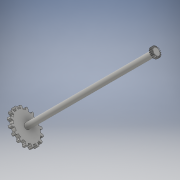
# Autodesk Inventor part: Connecting gears
Saved by Autodesk Inventor 2016 SP1 (Build 200210100, 210)
## iProperties
Created: 2016-02-23
Part Number: Connecting gears
Material: Generic
Document SubType Name: Modeling
Designer: Tore Den Store
Density: 1 g/cm^3
Appearance: Default
Author: Tore Den Store
Autodesk Inventor part; units mm, degrees
ref_plane "YZ Plane" through (0, 0, 0) normal (1, 0, 0) x (0, 1, 0)
ref_plane "XZ Plane" through (0, 0, 0) normal (0, 1, 0) x (-1, 0, 0)
ref_plane "XY Plane" through (0, 0, 0) normal (0, 0, 1) x (1, 0, 0)
sketch "Sketch1" plane through (0, 0, 0) normal (0, 1, 0) x (-1, 0, 0)
  circle A0 centre (0, 0) radius 100
  dimension "d0" = 200
  constraints: 1 centre point, 1 coincident
  measures "d0" diameter of A0
extrude "Extrusion1" add sketch "Sketch1" along normal blind 25
sketch "Sketch2" plane through (0, 25, 0) normal (0, 1, 0) x (1, 0, 0)
  circle A0 centre (0, 0) radius 100 projected
  line L0 (0, 0) -> (-99.5185, -9.8017)
  line L1 (0, 0) -> (-99.5185, 9.8017)
  line L2 (0, 0) -> (-100, 0) construction
  circle A1 centre (0, 0) radius 100 projected
  line L3 (0, 0) -> (100, 0) construction
  line L4 (-100, 0) -> (-120, 0)
  line L5 (-99.5185, 9.8017) -> (-109.5185, 9.8017)
  line L6 (-109.5185, 9.8017) -> (-120, 5.9868)
  line L7 (-120, 5.9868) -> (-120, 0)
  line L8 (-120, 0) -> (-120, -5.9868)
  line L9 (-120, -5.9868) -> (-109.5185, -9.8017)
  line L10 (-109.5185, -9.8017) -> (-99.5185, -9.8017)
  dimension "d3" = 11.25
  dimension "d4" = 180
  dimension "d5" = 5.625
  dimension "d8" = 110
  dimension "d9" = 110
  dimension "d10" = 10
  dimension "d11" = 10
  dimension "d12" = 20
  constraints: 22 end point, 3 horizontal, 2 point on circle, 1 collinear, 1 horizontal alignment, 1 parallel, 1 perpendicular, 1 vertical, 1 other
  measures "d3" angle of L0 L1
  measures "d4" angle of L2 L3
  measures "d5" angle of L0 L2
  measures "d8" angle of L6 L7
  measures "d9" angle of L9 L8
  measures "d10" distance of L9.end L0.end
  measures "d11" distance of L1.end L5.end
  measures "d12" distance of L2.end L4.end
extrude "Extrusion2" add sketch "Sketch2" against normal blind 25 contours A0 L4 L7 L6 L5 | L10 L9 L8 L4 A0
pattern_circular "Circular Pattern1" count 16 over 360 about axis through (0, 0, 0) along (0, 1, 0) of "Extrusion2"
sketch "Sketch3" plane through (0, 0, 0) normal (0, -1, 0) x (1, 0, 0)
  circle A0 centre (0, 0) radius 20
  dimension "d18" = 40
  constraints: 1 centre point, 1 coincident
  measures "d18" diameter of A0
extrude "Extrusion3" add sketch "Sketch3" along normal blind 925
sketch "Sketch4" plane through (0, -925, 0) normal (0, -1, 0) x (1, 0, 0)
  circle A0 centre (0, 0) radius 25
  dimension "d21" = 50
  constraints: 1 centre point, 1 coincident
  measures "d21" diameter of A0
extrude "Extrusion4" add sketch "Sketch4" along normal blind 20
sketch "Sketch5" plane through (0, -945, 0) normal (0, -1, 0) x (1, 0, 0)
  line L0 (0, 0) -> (-2.75, 24.9496) construction
  line L1 (0, 0) -> (0, 25) construction
  line L2 (0, 25) -> (0, 35) construction
  line L3 (-2, 24.9199) -> (-2, 31.9199)
  line L4 (-2, 31.9199) -> (-0.8789, 35)
  line L5 (0.8789, 35) -> (2, 31.9199)
  line L6 (2, 31.9199) -> (2, 24.9199)
  circle A0 centre (0, 0) radius 25 projected
  line L7 (-0.8789, 35) -> (0.8789, 35)
  dimension "d44" = 160
  dimension "d45" = 4
  dimension "d46" = 7
  dimension "d47" = 2
  dimension "d49" = 160
  dimension "d51" = 10
  constraints: 16 end point, 3 point on circle, 2 parallel, 2 vertical, 1 horizontal
  measures "d44" angle of L4 L3
  measures "d45" distance between parallel lines of L6 L3
  measures "d46" distance of L5.end L6.end
  measures "d47" distance between parallel lines of L2 L3
  measures "d49" angle of L6 L5
  measures "d51" distance from line of L1.end L7
extrude "Extrusion5" add sketch "Sketch5" against normal blind 20 contours L3 L4 L7 L5 L6 A0
pattern_circular "Circular Pattern2" count 20 over 360 about axis through (0, -925, 0) along (0, -1, 0) of "Extrusion5"
equation "\"d5\" = 0.5 * d3"
equation "\"d49\" = d44"
body "Solid1"
